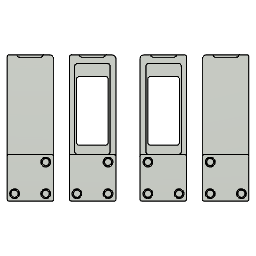
mriya-display-mcu-cover-v1.02 (Autodesk Fusion 360 design; units mm, degrees)
Autodesk Fusion 360 part; units mm, degrees
sketch "mriya-display-cover" plane through (0, 0, 0) normal (0, 0, 1) x (1, 0, 0)
  line L0 (-20.6, 56) -> (-8, 56)
  arc A0 (-5, 63) -> (-6.5, 64.5) centre (-6.5, 63) ccw construction
  line L1 (-48.5, 64.72) -> (-31.5, 64.72)
  line L2 (-44.4, 63.75) -> (-44.4, 64.72)
  line L3 (-43.6, 63.8) -> (-35, 63.8) construction
  line L4 (-48.5, 24.7) -> (-29.78, 24.7)
  line L5 (-44.4, 63.75) -> (-34.2, 63.75)
  arc A1 (-47.7, 64.5) -> (-48.5, 63.7) centre (-47.7, 63.7) ccw construction
  line L6 (-7.2, 61.3) -> (-7.2, 24.7)
  line L7 (-21.4, 61.3) -> (-7.2, 61.3)
  circle A2 centre (-20.5, 21.7) radius 1.7 construction
  line L8 (-23.5, 24.7) -> (-4.78, 24.7)
  circle A3 centre (-8, 21.7) radius 1.7 construction
  line L9 (-20.6, 28.5) -> (-20.6, 56)
  line L10 (-18.6, 63.8) -> (-10, 63.8) construction
  line L11 (-20.6, 28.5) -> (-8, 28.5)
  line L12 (-19.4, 63.75) -> (-9.2, 63.75)
  line L13 (-22.7, 64.5) -> (-6.5, 64.5) construction
  line L14 (-48.5, 6) -> (-48.5, 64.72)
  line L15 (-23.5, 6) -> (-4.78, 6)
  line L16 (-22.7, 6) -> (-5.8, 6) construction
  arc A4 (-48.5, 6.8) -> (-47.7, 6) centre (-47.7, 6.8) ccw construction
  circle A5 centre (-45.5, 9) radius 1.45
  arc A6 (-23.5, 6.8) -> (-22.7, 6) centre (-22.7, 6.8) ccw construction
  line L17 (-47.7, 6) -> (-30.8, 6) construction
  line L18 (-23.5, 6) -> (-23.5, 64.72)
  line L19 (-48.5, 6) -> (-29.78, 6)
  line L20 (-19.4, 63.75) -> (-19.4, 64.72)
  arc A7 (-22.7, 64.5) -> (-23.5, 63.7) centre (-22.7, 63.7) ccw construction
  line L21 (-23.5, 64.72) -> (-6.5, 64.72)
  line L22 (-21.4, 24.7) -> (-21.4, 61.3)
  circle A8 centre (-45.5, 21.7) radius 1.7 construction
  line L23 (-23.5, 6.8) -> (-23.5, 63.7) construction
  circle A9 centre (-33, 21.7) radius 1.7 construction
  line L24 (-47.7, 64.5) -> (-31.5, 64.5) construction
  circle A10 centre (-14.3, 15.5) radius 5 construction
  arc A11 (-30, 63) -> (-31.5, 64.5) centre (-31.5, 63) ccw construction
  line L25 (-8, 56) -> (-8, 28.5)
  line L26 (-29.78, 6) -> (-29.78, 63)
  line L27 (-48.5, 6.8) -> (-48.5, 63.7) construction
  arc A12 (-30.8, 6) -> (-30, 6.8) centre (-30.8, 6.8) ccw construction
  circle A13 centre (-20.5, 9) radius 1.45
  circle A14 centre (-33, 9) radius 1.45
  arc A15 (-5.8, 6) -> (-5, 6.8) centre (-5.8, 6.8) ccw construction
  circle A16 centre (-8, 9) radius 1.45
  line L28 (-4.78, 6) -> (-4.78, 63)
  line L29 (-5, 6.8) -> (-5, 63) construction
  line L30 (-30, 6.8) -> (-30, 63) construction
  circle A17 centre (-39.3, 15.5) radius 5 construction
  circle A18 centre (-39.3, 9) radius 1.5 construction
  circle A19 centre (-33, 21.7) radius 1.45
  circle A20 centre (-8, 21.7) radius 1.45
  circle A21 centre (-14.3, 9) radius 1.5 construction
  arc A22 (-44.3, 64.5) -> (-43.6, 63.8) centre (-43.6, 64.5) ccw construction
  arc A23 (-35, 63.8) -> (-34.3, 64.5) centre (-35, 64.5) ccw construction
  line L31 (-34.2, 64.75) -> (-34.2, 63.75)
  line L32 (-9.2, 64.75) -> (-9.2, 63.75)
  arc A24 (-19.3, 64.5) -> (-18.6, 63.8) centre (-18.6, 64.5) ccw construction
  arc A25 (-10, 63.8) -> (-9.3, 64.5) centre (-10, 64.5) ccw construction
  arc A26 (-4.78, 63) -> (-6.5, 64.72) centre (-6.5, 63) ccw
  arc A27 (-29.78, 63) -> (-31.5, 64.72) centre (-31.5, 63) ccw
  dimension "d523" = 2.9
  dimension "d524" = 2.9
  dimension "d525" = 10
  dimension "d526" = 3.4
  dimension "d527" = 3.4
  dimension "d530" = 2.9
  dimension "d531" = 2.9
  dimension "d532" = 10
  dimension "d533" = 3.4
  dimension "d534" = 3.4
  dimension "d558" = 3
  dimension "d559" = 2.9
  dimension "d560" = 2.9
  dimension "d562" = 3
  constraint perpendicular L13 L29
  constraint perpendicular L16 L23
  constraint tangent A6 L23
  constraint tangent L16 A6
  constraint tangent A15 L29
  constraint tangent L16 A15
  constraint tangent A7 L23
  constraint tangent L13 A7
  constraint tangent A0 L29
  constraint tangent A0 L13
  constraint perpendicular L9 L11
  constraint perpendicular L0 L9
  constraint perpendicular L11 L25
  constraint coincident L8.end L28
  constraint perpendicular L15 L28
  constraint perpendicular L18 L21
  constraint coincident L8.start L23
  constraint coincident L22.start L8
  constraint coincident L6.end L8
  constraint perpendicular L24 L30
  constraint perpendicular L17 L27
  constraint tangent A4 L27
  constraint tangent A4 L17
  constraint tangent A12 L30
  constraint tangent L17 A12
  constraint tangent A1 L27
  constraint tangent A1 L24
  constraint tangent A11 L30
  constraint tangent L24 A11
  constraint coincident L4.end L26
  constraint perpendicular L19 L26
  constraint perpendicular L1 L14
  constraint coincident L4.start L27
  constraint horizontal L12
  constraint coincident L20.end L21
  constraint perpendicular L20 L21
  constraint coincident L2.end L1
  constraint perpendicular L1 L2
  constraint concentric A9 A19
  constraint concentric A3 A20
  constraint tangent L3 A22
  constraint tangent L3 A23
  constraint perpendicular L5 L31
  constraint perpendicular L12 L32
  constraint tangent L10 A24
  constraint tangent L10 A25
  constraint tangent L21 A26
  constraint tangent L28 A26
  constraint tangent L1 A27
  constraint tangent L26 A27
  measures "d523" diameter of A13
  measures "d524" diameter of A16
  measures "d525" diameter of A10
  measures "d526" diameter of A2
  measures "d527" diameter of A3
  measures "d530" diameter of A5
  measures "d531" diameter of A14
  measures "d532" diameter of A17
  measures "d533" diameter of A8
  measures "d534" diameter of A9
  measures "d558" diameter of A18
  measures "d559" diameter of A19
  measures "d560" diameter of A20
  measures "d562" diameter of A21
extrude "Extrude71" add sketch "mriya-display-cover" along normal blind 6.6 contours L4 L14 L19 L26 | L8 L15 L18 L28 makes body 1 at (-42.6186, 18.7741, 0) makes body 2 at (-17.6186, 18.7741, 0)
extrude "Extrude72" add sketch "mriya-display-cover" along normal blind 3.6 contours L1 L2 L4 L5 L14 L26 L31 A27 | L6 L7 L8 L12 L18 L20 L21 L22 L28 L32 A26 bodies 1 2
extrude "Extrude73" add sketch "mriya-display-cover" along normal blind 1.6 contours L1 L2 L5 L31 | L12 L20 L21 L32 | A5 | A13 | A14 | A16 | A19 | A20 bodies 1 2
extrude "Extrude74" add sketch "mriya-display-cover" along normal blind 0.8 contours L6 L7 L8 L22 bodies 2
fillet "Fillet52" radius 0.8 10 edges at (-29.78, 6, 3.3) (-29.78, 24.7, 5.1) (-48.5, 6, 3.3) (-48.5, 24.7, 5.1) (-48.5, 64.72, 1.8) (-4.78, 6, 3.3) (-23.5, 6, 3.3) (-4.78, 24.7, 5.1) (-23.5, 24.7, 5.1) (-23.5, 64.72, 1.8) on bodies 1 2
fillet "Fillet57" radius 0.8 4 edges at (-44.4, 63.75, 2.6) (-34.2, 63.75, 2.6) (-9.2, 63.75, 2.6) (-19.4, 63.75, 2.6) on bodies 1 2
fillet "Fillet58" radius 0.6 4 edges at (-34.2, 64.72, 2.6) (-44.4, 64.72, 2.6) (-9.2, 64.72, 2.6) (-19.4, 64.72, 2.6) on bodies 1 2
fillet "Fillet59" radius 1 4 edges at (-20.6, 56, 0.4) (-8, 56, 0.4) (-8, 28.5, 0.4) (-20.6, 28.5, 0.4) on bodies 2
fillet "Fillet60" radius 1.2 4 edges at (-21.4, 61.3, 2.2) (-7.2, 61.3, 2.2) (-21.4, 24.7, 2.2) (-7.2, 24.7, 2.2) on bodies 2
chamfer "Chamfer25" distance 0.5 angle 45 6 edges at (-46.8519, 9.5243, 6.6) (-34.3519, 9.5243, 6.6) (-34.3519, 22.2243, 6.6) (-21.8519, 9.5243, 6.6) (-9.3519, 9.5243, 6.6) (-9.3519, 22.2243, 6.6) on bodies 1 2
mirror "Mirror8" about plane through (0, 0, 0) normal (1, 0, 0) of bodies 2 1 makes body 3 at (42.26, 44.5733, 0) makes body 4 at (12.4267, 14.0333, 0)
named bodies: "right-mcu", "right-display", "left-mcu", "left-display"
